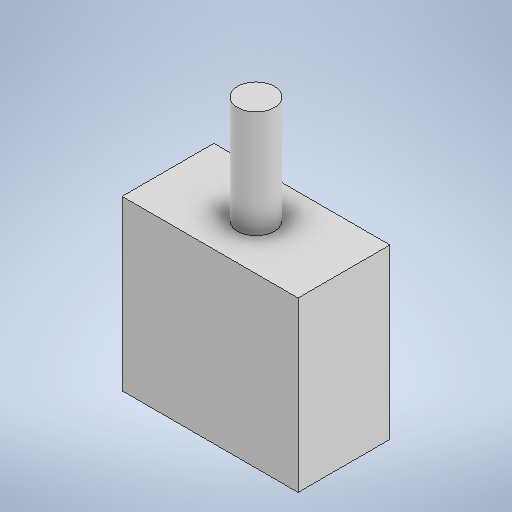
# Autodesk Inventor part: Servo_SG90
Saved by Autodesk Inventor 2025 (Build 290162000, 162)
## iProperties
Created: 2026-07-01
Part Number: Servo_SG90
Material: Generisch
Document SubType Name: Modeling
Designer: wavid
Mass: 6.32534 g
Surface Area: 23.3931 cm^2
Volume: 6.32534 cm^3
Density: 1 g/cm^3
Appearance: Vorgabe
Author: wavid
Autodesk Inventor part; units mm, degrees
ref_plane "YZ Plane" through (0, 0, 0) normal (1, 0, 0) x (0, 1, 0)
ref_plane "XZ Plane" through (0, 0, 0) normal (0, 1, 0) x (-1, 0, 0)
sketch "Skizze1" plane through (0, 0, 0) normal (0, 0, 1) x (1, 0, 0)
  line L0 (-11.5, -6) -> (11.5, -6)
  line L1 (11.5, -6) -> (11.5, 6)
  line L2 (11.5, 6) -> (-11.5, 6)
  line L3 (-11.5, 6) -> (-11.5, -6)
  constraints: 8 end point, 2 parallel, 1 horizontal, 1 perpendicular
extrude "Extrusion1" add sketch "Skizze1" along normal blind 22
ref_plane "Arbeitsebene1" through (0, 0, 22) normal (0, 0, 1) x (1, 0, 0)
sketch "Skizze2" plane through (0, 0, 22) normal (0, 0, 1) x (1, 0, 0)
  circle A0 centre (0, 0) radius 2.4
  constraints: 1 centre point
extrude "Extrusion2" add sketch "Skizze2" along normal blind 14 separate body
